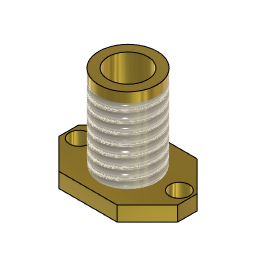
SMA Connector v2 (Autodesk Fusion 360 design; units mm, degrees)
Autodesk Fusion 360 part; units mm, degrees
sketch "Sketch1" plane through (0, 0, 0) normal (0, 0, 1) x (1, 0, 0)
  circle A0 centre (0, 0) radius 0.635
  dimension "d1" = 1.27
  constraint coincident A0.centre origin
  measures "d1" diameter of A0
extrude "Extrude1" add sketch "Sketch1" along normal blind 8 makes body 1
sketch "Sketch2" plane through (0, 0, 0) normal (0, 0, 1) x (1, 0, 0)
  circle A0 centre (0, 0) radius 0.635
  circle A1 centre (0, 0) radius 2
  dimension "d4" = 1.27
  dimension "d5" = 4
  constraint coincident A0.centre A1.centre
  constraint concentric A0 A1
  measures "d4" diameter of A0
  measures "d5" diameter of A1
extrude "Extrude2" add sketch "Sketch2" along normal blind 6 separate body contours A0 | A1 makes body 2
sketch "Sketch3" plane through (0, 0, 0) normal (0, 0, 1) x (1, 0, 0)
  circle A0 centre (0, 0) radius 2
  circle A1 centre (0, 0) radius 3.175
  dimension "d8" = 4
  dimension "d9" = 6.35
  constraint coincident A0.centre A1.centre
  constraint concentric A0 A1
  measures "d8" diameter of A0
  measures "d9" diameter of A1
extrude "Extrude3" add sketch "Sketch3" along normal blind 10 separate body makes body 3
sketch "Sketch4" plane through (0, 0, 0) normal (0, 0, 1) x (1, 0, 0)
  line L0 (-6.0124, 0.9876) -> (-2.9509, 4.0491)
  line L1 (-2.9509, 4.0491) -> (2.9509, 4.0491)
  line L2 (2.9509, 4.0491) -> (6.0124, 0.9876)
  line L3 (6.0124, 0.9876) -> (6.0124, -0.9876)
  line L4 (6.0124, -0.9876) -> (2.9509, -4.0491)
  line L5 (2.9509, -4.0491) -> (-2.9509, -4.0491)
  line L6 (-2.9509, -4.0491) -> (-6.0124, -0.9876)
  line L7 (-6.0124, -0.9876) -> (-6.0124, 0.9876)
  constraint horizontal L1
  constraint perpendicular L0 L2
  constraint perpendicular L1 L3
  constraint perpendicular L3 L5
  constraint perpendicular L5 L7
  constraint equal L3 L7
  constraint equal L1 L5
  constraint equal L0 L2
  constraint equal L4 L6
extrude "Extrude4" add sketch "Sketch4" along normal blind 1.5 separate body makes body 4
hole "Hole1" at (4.8124, 0.3886, 1.5) direction (0, 0, -1) diameter 2 depth 2 tip angle 118 bodies 4
hole "Hole2" at (-4.8124, -0.1187, 1.5) direction (0, 0, -1) diameter 2 depth 2 tip angle 118 bodies 4
extrude "Extrude5" add 1 faces at (0.4074, -0.1723, 0) along direction (0, 0, -1) blind 0.5 separate body on bodies 1 makes body 5
extrude "Extrude6" add 1 faces at (0.637, 0.1965, 0) along direction (0, 0, -1) blind 0.5 separate body on bodies 2 makes body 6
hole "Hole3" at (0, 0, 8) direction (0, 0, -1) diameter 0.5 depth 6 tip angle 118 bodies 1 2
thread "Thread2" "ISO Metric profile 6.0 M6x1 M6x1 6g" major diameter 5.884 minor diameter 4.7435 pitch 1 angle 60 resizes the face on face at (3.1711, -0.1583, 6.6667) from (0, 0, 0) to (0, 0, 9) on bodies 3
named bodies: "Center Pin", "Dielectric", "Outer body"
